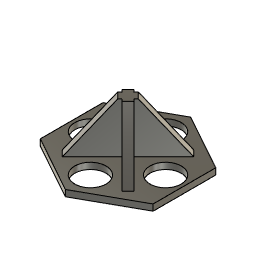
conductive_015_hexagon_tight (Autodesk Fusion 360 design; units mm, degrees)
Autodesk Fusion 360 part; units mm, degrees
other "Base Mesh Feature1"
sketch "Sketch1" plane through (0, 0, 0) normal (0, 0, 1) x (1, 0, 0)
  circle A0 centre (0, 0) radius 1
  line L0 (0, 0) -> (20, 20) construction
  dimension "d1" = 2
  constraint coincident A0.centre L0.start
  measures "d1" diameter of A0
other "Modify1"
sketch "Sketch2" plane through (0, 0, 0) normal (0, 0, 1) x (1, 0, 0)
  line L0 (18, -10) -> (18, 10)
  line L1 (-18, 10) -> (-18, -10)
  line L2 (0, 20) -> (-18, 10)
  line L3 (0, 20) -> (18, 10)
  line L4 (18, -10) -> (0, -20)
  line L5 (-18, -10) -> (0, -20)
  circle A0 centre (0, 12) radius 5
  circle A1 centre (-12, 0) radius 5
  circle A2 centre (0, -12) radius 5
  circle A3 centre (12, 0) radius 5
  dimension "d3" = 360
  constraint vertical L0
  constraint vertical L1
  constraint parallel L2 L4
  constraint parallel L3 L5
extrude "Extrude1" add sketch "Sketch2" along normal blind 2 makes body 1
ref_plane "WorkPlane1" through (10, 10, 0) normal (0.707107, -0.707107, 0) x (0.707107, 0.707107, 0)
sketch "Sketch3" plane through (0, 0, 0) normal (0.707107, -0.707107, 0) x (0.707107, 0.707107, 0)
  line L0 (-15, 2) -> (0, 2)
  line L1 (0, 18) -> (-2.3172, 18)
  line L2 (-2.3172, 18) -> (-14.8339, 2)
  line L3 (2.3172, 18) -> (14.8339, 2)
  line L4 (0, 18) -> (2.3172, 18)
  line L5 (15, 2) -> (0, 2)
  constraint horizontal L0
  constraint horizontal L1
  constraint coincident L0 L2.end
extrude "Extrude2" add sketch "Sketch3" along normal mid plane 2.72 separate body makes body 2
copy_body "CopyPasteBodies1" bodies 2 makes body 3
move_body "Move1" bodies 3 to x (0, -1, 0) y (1, 0, 0) z (0, 0, 1) at (0, 0, 0)
combine "Combine1" operation add target body 2 tool bodies 3 1
